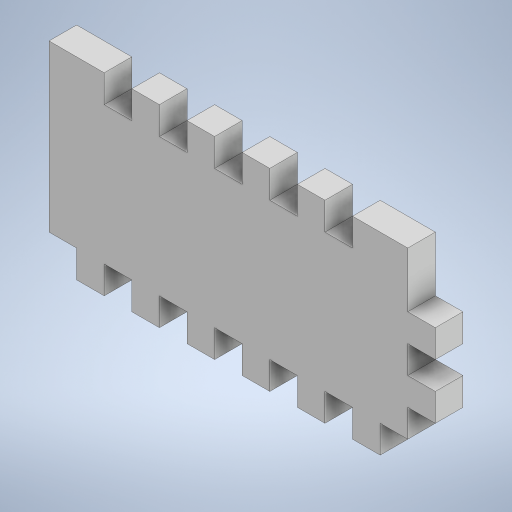
# Autodesk Inventor part: backside
Saved by Autodesk Inventor 2024 (Build 280153000, 153)
## iProperties
Created: 2024-04-15
Part Number: backside
Material: Generic
Document SubType Name: Modeling
Designer: srika
Density: 1 g/cm^3
Appearance: Default
Author: srika
Autodesk Inventor part; units mm, degrees
ref_plane "YZ Plane" through (0, 0, 0) normal (1, 0, 0) x (0, 1, 0)
ref_plane "XZ Plane" through (0, 0, 0) normal (0, 1, 0) x (-1, 0, 0)
ref_plane "XY Plane" through (0, 0, 0) normal (0, 0, 1) x (1, 0, 0)
sketch "Sketch2" plane through (0, 0, 0) normal (0, 0, 1) x (1, 0, 0)
  line L0 (0, 0) -> (5, 0)
  line L1 (5, 0) -> (5, 5)
  line L2 (5, 5) -> (0, 5)
  line L3 (0, 5) -> (0, 0)
  line L4 (0, 5) -> (65, 5)
  line L5 (65, 5) -> (65, 30)
  line L6 (65, 30) -> (0, 30)
  line L7 (0, 30) -> (0, 5)
  line L8 (10, 0) -> (15, 0)
  line L9 (15, 0) -> (15, 5)
  line L10 (10, 5) -> (10, 0)
  line L11 (20, 0) -> (25, 0)
  line L12 (25, 0) -> (25, 5)
  line L13 (20, 5) -> (20, 0)
  line L14 (30, 0) -> (35, 0)
  line L15 (35, 0) -> (35, 5)
  line L16 (30, 5) -> (30, 0)
  line L17 (40, 0) -> (45, 0)
  line L18 (45, 0) -> (45, 5)
  line L19 (40, 5) -> (40, 0)
  line L20 (50, 0) -> (55, 0)
  line L21 (55, 0) -> (55, 5)
  line L22 (50, 5) -> (50, 0)
  line L23 (60, 0) -> (65, 0)
  line L24 (65, 0) -> (65, 5)
  line L25 (60, 5) -> (60, 0)
  line L26 (65, 25) -> (70, 25)
  line L27 (70, 25) -> (70, 20)
  line L28 (70, 20) -> (65, 20)
  line L29 (65, 20) -> (65, 25)
  line L30 (65, 15) -> (70, 15)
  line L31 (70, 15) -> (70, 10)
  line L32 (70, 10) -> (65, 10)
  line L33 (65, 10) -> (65, 15)
  line L34 (0, 35) -> (5, 35)
  line L35 (5, 35) -> (5, 30)
  line L36 (5, 30) -> (0, 30)
  line L37 (0, 30) -> (0, 35)
  line L38 (15, 35) -> (15, 30)
  line L39 (15, 30) -> (10, 30)
  line L40 (10, 35) -> (15, 35)
  line L41 (10, 30) -> (10, 35)
  line L42 (25, 35) -> (25, 30)
  line L43 (25, 30) -> (20, 30)
  line L44 (20, 35) -> (25, 35)
  line L45 (20, 30) -> (20, 35)
  line L46 (35, 35) -> (35, 30)
  line L47 (35, 30) -> (30, 30)
  line L48 (30, 35) -> (35, 35)
  line L49 (30, 30) -> (30, 35)
  line L50 (45, 35) -> (45, 30)
  line L51 (45, 30) -> (40, 30)
  line L52 (40, 35) -> (45, 35)
  line L53 (40, 30) -> (40, 35)
  line L54 (55, 35) -> (55, 30)
  line L55 (55, 30) -> (50, 30)
  line L56 (50, 35) -> (55, 35)
  line L57 (50, 30) -> (50, 35)
  line L58 (65, 35) -> (65, 30)
  line L59 (65, 30) -> (60, 30)
  line L60 (60, 35) -> (65, 35)
  line L61 (60, 30) -> (60, 35)
  line L62 (-5, 35) -> (0, 35)
  line L63 (0, 35) -> (0, 0)
  line L64 (0, 0) -> (-5, 0)
  line L65 (-5, 0) -> (-5, 35)
  line L66 (-5, 5) -> (0, 5)
  line L67 (0, 5) -> (0, 0)
  line L68 (0, 0) -> (-5, 0)
  line L69 (-5, 0) -> (-5, 5)
  line L70 (55, 35) -> (60, 35)
  line L71 (60, 35) -> (60, 30)
  line L72 (60, 30) -> (55, 30)
  line L73 (55, 30) -> (55, 35)
  line L74 (60, 25) -> (65, 25)
  line L75 (65, 25) -> (65, 20)
  line L76 (65, 20) -> (60, 20)
  line L77 (60, 20) -> (60, 25)
  line L78 (60, 15) -> (65, 15)
  line L79 (65, 15) -> (65, 10)
  line L80 (65, 10) -> (60, 10)
  line L81 (60, 10) -> (60, 15)
  line L82 (60, 30) -> (65, 30)
  line L83 (65, 30) -> (65, 5)
  line L84 (65, 5) -> (60, 5)
  line L85 (60, 5) -> (60, 30)
  dimension "d97" = 10
  dimension "d102" = 25
  dimension "d105" = 10
  constraints: 172 end point, 22 parallel, 13 horizontal, 11 perpendicular, 6 point on line, 96 other
  measures "d97" distance of L0.start L8.start
  measures "d102" distance of L4.end L5.end
  measures "d105" distance of L6.end point (10, 30)
extrude "Extrusion3" add sketch "Sketch2" along normal blind 5 contours L3 L2 L1 L0 | L7 L6 L85 L77 L81 L4 L2 | L66 L65 L62 L37 L7 | L37 L34 L35 L6 | L4 L9 L8 L10 | L41 L40 L38 L6 | L4 L12 L11 L13 | L45 L44 L42 L6 | L4 L15 L14 L16 | L49 L48 L46 L6 | L4 L18 L17 L19 | L53 L52 L50 L6 | L4 L21 L20 L22 | L57 L56 L54 L6 | L54 L70 L61 L6 | L81 L78 L5 L80 | L74 L5 L76 L77
body "Solid3"
